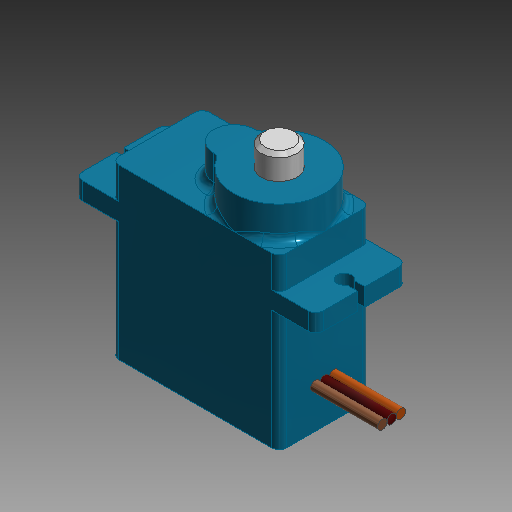
# Autodesk Inventor part: SG90
Saved by Autodesk Inventor 2019.2 (Build 232265000, 265)
## iProperties
Part Number: SG90
Material: ABS Plastic
Document SubType Name: Modeling
Designer: richard.girt
Mass: 7.54185 g
Surface Area: 27.447 cm^2
Volume: 7.11495 cm^3
Density: 1.06 g/cm^3
Appearance: Smooth - White
Author: richard.girt
Autodesk Inventor part; units mm, degrees
ref_plane "YZ Plane" through (0, 0, 0) normal (1, 0, 0) x (0, 1, 0)
ref_plane "XZ Plane" through (0, 0, 0) normal (0, 1, 0) x (-1, 0, 0)
ref_plane "XY Plane" through (0, 0, 0) normal (0, 0, 1) x (1, 0, 0)
sketch "Sketch1" plane through (0, 0, 0) normal (0, 1, 0) x (-1, 0, 0)
  line L0 (-11.25, -6.1) -> (11.25, -6.1)
  line L1 (11.25, -6.1) -> (11.25, 6.1)
  line L2 (11.25, 6.1) -> (-11.25, 6.1)
  line L3 (-11.25, 6.1) -> (-11.25, -6.1)
  line L4 (-11.25, -6.1) -> (11.25, 6.1) construction
  line L5 (11.25, -6.1) -> (-11.25, 6.1) construction
  point P0 (0, 0)
  dimension "d0" = 22.5
  dimension "d1" = 12.2
  constraints: 12 end point, 2 midpoint, 2 parallel, 1 horizontal, 1 perpendicular
  measures "d0" distance of L1.end L2.end
  measures "d1" distance of L2.end L0.start
extrude "Extrusion1" add sketch "Sketch1" against normal blind 16
sketch "Sketch2" plane through (0, 0, 0) normal (0, 1, 0) x (1, 0, 0)
  line L0 (16.15, -6.1) -> (-16.15, -6.1)
  line L1 (-16.15, -6.1) -> (-16.15, 6.1)
  line L2 (-16.15, 6.1) -> (16.15, 6.1)
  line L3 (16.15, 6.1) -> (16.15, -6.1)
  line L4 (16.15, -6.1) -> (-16.15, 6.1) construction
  line L5 (-16.15, -6.1) -> (16.15, 6.1) construction
  point P0 (-11.25, 6.1)
  point P1 (0, 0)
  dimension "d4" = 32.3
  constraints: 12 end point, 2 midpoint, 2 parallel, 1 horizontal, 1 perpendicular, 1 point on line
  measures "d4" distance of L0.start L0.end
extrude "Extrusion2" add sketch "Sketch2" along normal blind 2.36
sketch "Sketch3" plane through (0, 2.36, 0) normal (0, 1, 0) x (1, 0, 0)
  line L0 (-11.25, 6.1) -> (11.25, 6.1) construction
  line L1 (11.25, 6.1) -> (11.25, -6.1) construction
  line L2 (11.25, -6.1) -> (-11.25, -6.1) construction
  line L3 (-11.25, -6.1) -> (-11.25, 6.1) construction
  line L4 (-11.25, -6.1) -> (11.25, -6.1)
  line L5 (11.25, -6.1) -> (11.25, 6.1)
  line L6 (11.25, 6.1) -> (-11.25, 6.1)
  line L7 (-11.25, 6.1) -> (-11.25, -6.1)
  line L8 (-11.25, -6.1) -> (11.25, 6.1) construction
  line L9 (11.25, -6.1) -> (-11.25, 6.1) construction
  point P0 (0, 0)
  constraints: 12 end point, 2 midpoint, 2 parallel, 1 horizontal, 1 perpendicular
extrude "Extrusion3" add sketch "Sketch3" along normal blind 4.25
sketch "Sketch4" plane through (0, 6.61, 0) normal (0, 1, 0) x (1, 0, 0)
  line L0 (11.25, -6.1) -> (11.25, 6.1) construction
  line L1 (11.25, 6.1) -> (-11.25, 6.1) construction
  line L2 (-11.25, -6.1) -> (11.25, -6.1) construction
  circle A0 centre (5.15, 0) radius 6.1
  circle A1 centre (-0.85, 0) radius 2.75
  point P0 (0, 0)
  dimension "d9" = 5.5
  dimension "d10" = 6
  constraints: 3 tangent, 2 centre point, 1 horizontal alignment
  measures "d9" diameter of A1
  measures "d10" distance of A1.centre A0.centre
extrude "Extrusion4" add sketch "Sketch4" along normal blind 4.4
sketch "Sketch5" plane through (0, 11.01, 0) normal (0, 1, 0) x (1, 0, 0)
  arc A0 (-0.3206, -2.6986) -> (-0.3206, 2.6986) centre (5.15, 0) ccw construction
  circle A1 centre (5.15, 0) radius 2.4
  point P0 (0, 0)
  dimension "d13" = 4.8
  constraints: 1 centre point, 1 coincident
  measures "d13" diameter of A1
extrude "Extrusion5" add sketch "Sketch5" along normal blind 3.26 separate body
chamfer "Chamfer1" distance 0.5 angle 45 1 edges at (2.75, 14.27, 0)
sketch "Sketch6" plane through (0, 2.36, 0) normal (0, 1, 0) x (1, 0, 0)
  line L0 (-16.15, 6.1) -> (-16.15, -6.1) construction
  line L1 (-13.9, 0) -> (13.9, 0) construction
  circle A0 centre (-13.9, 0) radius 1
  circle A1 centre (13.9, 0) radius 1
  line L2 (-14.766, 0.5) -> (-16.15, 0.5)
  line L3 (-16.15, 0.5) -> (-16.15, -0.5)
  line L4 (-16.15, -0.5) -> (-14.766, -0.5)
  line L5 (-14.766, -0.5) -> (-14.766, 0.5)
  line L6 (-14.766, 0.5) -> (-16.15, -0.5) construction
  line L7 (-16.15, 0.5) -> (-14.766, -0.5) construction
  line L8 (16.15, 6.1) -> (16.15, -6.1) construction
  line L9 (14.766, -0.5) -> (16.15, -0.5)
  line L10 (16.15, -0.5) -> (16.15, 0.5)
  line L11 (16.15, 0.5) -> (14.766, 0.5)
  line L12 (14.766, 0.5) -> (14.766, -0.5)
  line L13 (14.766, -0.5) -> (16.15, 0.5) construction
  line L14 (16.15, -0.5) -> (14.766, 0.5) construction
  point P0 (0, 0)
  point P1 (0, 0)
  point P2 (-15.458, 0)
  point P3 (15.458, 0)
  dimension "d19" = 27.8
  dimension "d20" = 2
  dimension "d21" = 1
  constraints: 26 end point, 5 midpoint, 5 parallel, 4 point on circle, 3 coincident, 3 horizontal, 2 centre point, 2 perpendicular, 2 point on line, 1 equal radius
  measures "d19" distance of L1.start L1.end
  measures "d20" diameter of A0
  measures "d21" distance between parallel lines of L4 L2
extrude "Extrusion6" cut sketch "Sketch6" against normal through all bodies 1
fillet "Fillet1" radius 1 19 edges at (11.25, 4.485, 6.1) (11.25, 4.485, -6.1) (11.25, -8, 6.1) (11.25, -8, -6.1) (-11.25, 4.485, 6.1) (-11.25, -8, 6.1) (-11.25, 4.485, -6.1) (-11.25, -8, -6.1) (16.15, 1.18, -6.1) (16.15, 1.18, 6.1) (-16.15, 1.18, -6.1) (-16.15, 1.18, 6.1) (-0.3206, 8.81, 2.6986) (-0.3206, 8.81, -2.6986) (1.9291, 6.61, -5.1803) (-3.6, 6.61, 0) (1.9291, 6.61, 5.1803) (9.4634, 6.61, 4.3134) (9.4634, 6.61, -4.3134)
sketch "Sketch7" plane through (11.25, -16, -5.1) normal (1, 0, 0) x (0, 0, -1)
  line L0 (0, 16) -> (0, 0) construction
  line L1 (0, 0) -> (-10.2, 0) construction
  line L2 (-10.2, 16) -> (-10.2, 0) construction
  line L3 (-10.2, 5.3) -> (0, 5.3) construction
  circle A0 centre (-5.1, 5.3) radius 0.625
  circle A1 centre (-3.85, 5.3) radius 0.625
  circle A2 centre (-6.35, 5.3) radius 0.625
  point P0 (-5.1, 16)
  dimension "d25" = 5.3
  dimension "d26" = 1.25
  constraints: 4 equal radius, 4 point on line, 3 centre point, 2 end point, 1 midpoint, 1 perpendicular
  measures "d25" distance between parallel lines of L3 L1
  measures "d26" diameter of A1
extrude "Extrusion7" add sketch "Sketch7" along normal blind 9 separate body
body "Solid1"
body "Solid2"
body "Solid3"
